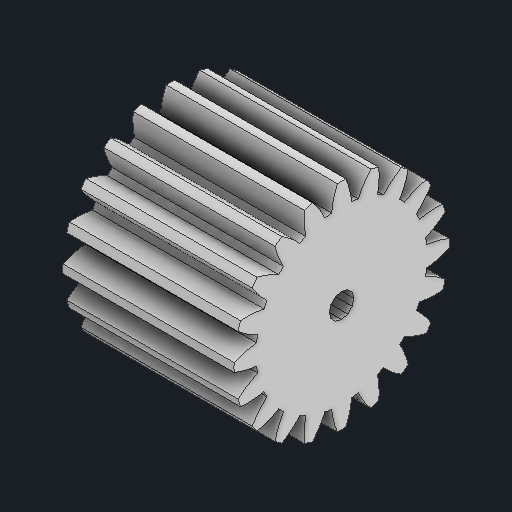
# Autodesk Inventor part: gear base
Saved by Autodesk Inventor 2024 (Build 280153000, 153)
## iProperties
Created: 2023-06-18
Part Number: gear base
Material: 일반
Document SubType Name: Modeling
Designer: 6gioc
Density: 1 g/cm^3
Appearance: 기본값
Mass: 18.4173 g
Surface Area: 64.8301 cm^2
Volume: 18.4173 cm^3
Author: 6gioc
Autodesk Inventor part; units mm, degrees
ref_plane "YZ Plane" through (0, 0, 0) normal (1, 0, 0) x (0, 1, 0)
ref_plane "XZ Plane" through (0, 0, 0) normal (0, 1, 0) x (-1, 0, 0)
ref_plane "XY Plane" through (0, 0, 0) normal (0, 0, 1) x (1, 0, 0)
sketch "스케치1" plane through (0, 0, 0) normal (1, 0, 0) x (0, 1, 0)
  circle A0 centre (0, 0) radius 22.155
  circle A1 centre (0, 0) radius 2.5
  line L0 (2.5, 0) -> (2.1651, -1.25)
  line L1 (2.1651, -1.25) -> (1.25, -2.1651)
  line L2 (1.25, -2.1651) -> (0, -2.5)
  line L3 (0, -2.5) -> (-1.25, -2.1651)
  line L4 (-1.25, -2.1651) -> (-2.1651, -1.25)
  line L5 (-2.1651, -1.25) -> (-2.5, 0)
  line L6 (-2.5, 0) -> (-2.1651, 1.25)
  line L7 (-2.1651, 1.25) -> (-1.25, 2.1651)
  line L8 (-1.25, 2.1651) -> (0, 2.5)
  line L9 (0, 2.5) -> (1.25, 2.1651)
  line L10 (1.25, 2.1651) -> (2.1651, 1.25)
  line L11 (2.1651, 1.25) -> (2.5, 0)
  dimension "d4" = 5
  dimension "d0" = 44.31
  constraints: 24 end point, 4 coincident, 1 centre point, 1 horizontal alignment, 27 other
  measures "d0" diameter of A0
extrude "돌출1" add sketch "스케치1" along normal blind 15 contours A0 | L11 A1 | A1 L0 | L10 A1 | A1 L1 | L9 A1 | A1 L2 | L8 A1 | A1 L3 | L7 A1 | A1 L4 | L6 A1 | A1 L5
spur gear teeth "스퍼 기어1" teeth 20 pitch diameter 40 tip diameter 44 root diameter 35 face width 15 trims to tip circle yes start plane through (15, 0, 0) normal (1, 0, 0) x (0, 1, 0)
sketch "스케치2" plane through (0, 0, 0) normal (-1, 0, 0) x (0, 0, 1)
  arc A0 (18.2923, 12.2225) -> (17.277, 13.6201) centre (0, 0) ccw projected
  arc A1 (17.277, 13.6201) -> (12.8506, 11.879) centre (21.0695, -2.5188) ccw projected
  arc A2 (12.8506, 11.879) -> (11.879, 12.8506) centre (0, 0) ccw projected
  arc A3 (11.879, 12.8506) -> (13.6201, 17.277) centre (-2.5188, 21.0695) ccw projected
  arc A4 (13.6201, 17.277) -> (12.2225, 18.2923) centre (0, 0) ccw projected
  arc A5 (12.2225, 18.2923) -> (8.5509, 15.2687) centre (20.8166, 4.1153) ccw projected
  arc A6 (8.5509, 15.2687) -> (7.3265, 15.8925) centre (0, 0) ccw projected
  arc A7 (7.3265, 15.8925) -> (7.6146, 20.6402) centre (-8.9064, 19.2599) ccw projected
  arc A8 (7.6146, 20.6402) -> (5.9717, 21.174) centre (0, 0) ccw projected
  arc A9 (5.9717, 21.174) -> (3.4141, 17.1637) centre (18.5261, 10.3466) ccw projected
  arc A10 (3.4141, 17.1637) -> (2.0569, 17.3787) centre (0, 0) ccw projected
  arc A11 (2.0569, 17.3787) -> (0.8637, 21.983) centre (-14.4221, 15.565) ccw projected
  arc A12 (0.8637, 21.983) -> (-0.8637, 21.983) centre (0, 0) ccw projected
  arc A13 (-0.8637, 21.983) -> (-2.0569, 17.3787) centre (14.4221, 15.565) ccw projected
  arc A14 (-2.0569, 17.3787) -> (-3.4141, 17.1637) centre (0, 0) ccw projected
  arc A15 (-3.4141, 17.1637) -> (-5.9717, 21.174) centre (-18.5261, 10.3466) ccw projected
  arc A16 (-5.9717, 21.174) -> (-7.6146, 20.6402) centre (0, 0) ccw projected
  arc A17 (-7.6146, 20.6402) -> (-7.3265, 15.8925) centre (8.9064, 19.2599) ccw projected
  arc A18 (-7.3265, 15.8925) -> (-8.5509, 15.2687) centre (0, 0) ccw projected
  arc A19 (-8.5509, 15.2687) -> (-12.2225, 18.2923) centre (-20.8166, 4.1153) ccw projected
  arc A20 (-12.2225, 18.2923) -> (-13.6201, 17.277) centre (0, 0) ccw projected
  arc A21 (-13.6201, 17.277) -> (-11.879, 12.8506) centre (2.5188, 21.0695) ccw projected
  arc A22 (-11.879, 12.8506) -> (-12.8506, 11.879) centre (0, 0) ccw projected
  arc A23 (-12.8506, 11.879) -> (-17.277, 13.6201) centre (-21.0695, -2.5188) ccw projected
  arc A24 (-17.277, 13.6201) -> (-18.2923, 12.2225) centre (0, 0) ccw projected
  arc A25 (-18.2923, 12.2225) -> (-15.2687, 8.5509) centre (-4.1153, 20.8166) ccw projected
  arc A26 (-15.2687, 8.5509) -> (-15.8925, 7.3265) centre (0, 0) ccw projected
  arc A27 (-15.8925, 7.3265) -> (-20.6402, 7.6146) centre (-19.2599, -8.9064) ccw projected
  arc A28 (-20.6402, 7.6146) -> (-21.174, 5.9717) centre (0, 0) ccw projected
  arc A29 (-21.174, 5.9717) -> (-17.1637, 3.4141) centre (-10.3466, 18.5261) ccw projected
  arc A30 (-17.1637, 3.4141) -> (-17.3787, 2.0569) centre (0, 0) ccw projected
  arc A31 (-17.3787, 2.0569) -> (-21.983, 0.8637) centre (-15.565, -14.4221) ccw projected
  arc A32 (-21.983, 0.8637) -> (-21.983, -0.8637) centre (0, 0) ccw projected
  arc A33 (-21.983, -0.8637) -> (-17.3787, -2.0569) centre (-15.565, 14.4221) ccw projected
  arc A34 (-17.3787, -2.0569) -> (-17.1637, -3.4141) centre (0, 0) ccw projected
  arc A35 (-17.1637, -3.4141) -> (-21.174, -5.9717) centre (-10.3466, -18.5261) ccw projected
  arc A36 (-21.174, -5.9717) -> (-20.6402, -7.6146) centre (0, 0) ccw projected
  arc A37 (-20.6402, -7.6146) -> (-15.8925, -7.3265) centre (-19.2599, 8.9064) ccw projected
  arc A38 (-15.8925, -7.3265) -> (-15.2687, -8.5509) centre (0, 0) ccw projected
  arc A39 (-15.2687, -8.5509) -> (-18.2923, -12.2225) centre (-4.1153, -20.8166) ccw projected
  arc A40 (-18.2923, -12.2225) -> (-17.277, -13.6201) centre (0, 0) ccw projected
  arc A41 (-17.277, -13.6201) -> (-12.8506, -11.879) centre (-21.0695, 2.5188) ccw projected
  arc A42 (-12.8506, -11.879) -> (-11.879, -12.8506) centre (0, 0) ccw projected
  arc A43 (-11.879, -12.8506) -> (-13.6201, -17.277) centre (2.5188, -21.0695) ccw projected
  arc A44 (-13.6201, -17.277) -> (-12.2225, -18.2923) centre (0, 0) ccw projected
  arc A45 (-12.2225, -18.2923) -> (-8.5509, -15.2687) centre (-20.8166, -4.1153) ccw projected
  arc A46 (-8.5509, -15.2687) -> (-7.3265, -15.8925) centre (0, 0) ccw projected
  arc A47 (-7.3265, -15.8925) -> (-7.6146, -20.6402) centre (8.9064, -19.2599) ccw projected
  arc A48 (-7.6146, -20.6402) -> (-5.9717, -21.174) centre (0, 0) ccw projected
  arc A49 (-5.9717, -21.174) -> (-3.4141, -17.1637) centre (-18.5261, -10.3466) ccw projected
  arc A50 (-3.4141, -17.1637) -> (-2.0569, -17.3787) centre (0, 0) ccw projected
  arc A51 (-2.0569, -17.3787) -> (-0.8637, -21.983) centre (14.4221, -15.565) ccw projected
  arc A52 (-0.8637, -21.983) -> (0.8637, -21.983) centre (0, 0) ccw projected
  arc A53 (0.8637, -21.983) -> (2.0569, -17.3787) centre (-14.4221, -15.565) ccw projected
  arc A54 (2.0569, -17.3787) -> (3.4141, -17.1637) centre (0, 0) ccw projected
  arc A55 (3.4141, -17.1637) -> (5.9717, -21.174) centre (18.5261, -10.3466) ccw projected
  arc A56 (5.9717, -21.174) -> (7.6146, -20.6402) centre (0, 0) ccw projected
  arc A57 (7.6146, -20.6402) -> (7.3265, -15.8925) centre (-8.9064, -19.2599) ccw projected
  arc A58 (7.3265, -15.8925) -> (8.5509, -15.2687) centre (0, 0) ccw projected
  arc A59 (8.5509, -15.2687) -> (12.2225, -18.2923) centre (20.8166, -4.1153) ccw projected
  arc A60 (12.2225, -18.2923) -> (13.6201, -17.277) centre (0, 0) ccw projected
  arc A61 (13.6201, -17.277) -> (11.879, -12.8506) centre (-2.5188, -21.0695) ccw projected
  arc A62 (11.879, -12.8506) -> (12.8506, -11.879) centre (0, 0) ccw projected
  arc A63 (12.8506, -11.879) -> (17.277, -13.6201) centre (21.0695, 2.5188) ccw projected
  arc A64 (17.277, -13.6201) -> (18.2923, -12.2225) centre (0, 0) ccw projected
  arc A65 (18.2923, -12.2225) -> (15.2687, -8.5509) centre (4.1153, -20.8166) ccw projected
  arc A66 (15.2687, -8.5509) -> (15.8925, -7.3265) centre (0, 0) ccw projected
  arc A67 (15.8925, -7.3265) -> (20.6402, -7.6146) centre (19.2599, 8.9064) ccw projected
  arc A68 (20.6402, -7.6146) -> (21.174, -5.9717) centre (0, 0) ccw projected
  arc A69 (21.174, -5.9717) -> (17.1637, -3.4141) centre (10.3466, -18.5261) ccw projected
  arc A70 (17.1637, -3.4141) -> (17.3787, -2.0569) centre (0, 0) ccw projected
  arc A71 (17.3787, -2.0569) -> (21.983, -0.8637) centre (15.565, 14.4221) ccw projected
  arc A72 (21.983, -0.8637) -> (21.983, 0.8637) centre (0, 0) ccw projected
  arc A73 (21.983, 0.8637) -> (17.3787, 2.0569) centre (15.565, -14.4221) ccw projected
  arc A74 (17.3787, 2.0569) -> (17.1637, 3.4141) centre (0, 0) ccw projected
  arc A75 (17.1637, 3.4141) -> (21.174, 5.9717) centre (10.3466, 18.5261) ccw projected
  arc A76 (21.174, 5.9717) -> (20.6402, 7.6146) centre (0, 0) ccw projected
  arc A77 (20.6402, 7.6146) -> (15.8925, 7.3265) centre (19.2599, -8.9064) ccw projected
  arc A78 (15.8925, 7.3265) -> (15.2687, 8.5509) centre (0, 0) ccw projected
  arc A79 (15.2687, 8.5509) -> (18.2923, 12.2225) centre (4.1153, 20.8166) ccw projected
  line L0 (1.25, 2.1651) -> (0, 2.5) projected
  line L1 (2.1651, 1.25) -> (1.25, 2.1651) projected
  line L2 (2.5, 0) -> (2.1651, 1.25) projected
  line L3 (2.1651, -1.25) -> (2.5, 0) projected
  line L4 (1.25, -2.1651) -> (2.1651, -1.25) projected
  line L5 (0, -2.5) -> (1.25, -2.1651) projected
  line L6 (-1.25, -2.1651) -> (0, -2.5) projected
  line L7 (-2.1651, -1.25) -> (-1.25, -2.1651) projected
  line L8 (-2.5, 0) -> (-2.1651, -1.25) projected
  line L9 (-2.1651, 1.25) -> (-2.5, 0) projected
  line L10 (-1.25, 2.1651) -> (-2.1651, 1.25) projected
  line L11 (0, 2.5) -> (-1.25, 2.1651) projected
extrude "돌출2" add sketch "스케치2" along normal blind 20
